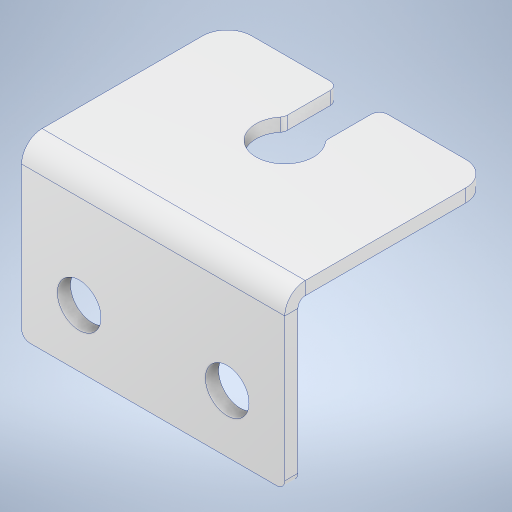
# Autodesk Inventor part: Door Stop
Saved by Autodesk Inventor 2024 (Build 280153000, 153)
## iProperties
Created: 2023-06-16
Part Number: Door Stop
Material: Aluminum 6061
Document SubType Name: Sheet Metal
Designer: Ishaan
Density: 2.7 g/cm^3
Appearance: Aluminum - Flat
Sheet Metal Rule: SendCutSend_Alu_1-16
Author: Ishaan
Autodesk Inventor part; units mm, degrees
ref_plane "YZ Plane" through (0, 0, 0) normal (1, 0, 0) x (0, 1, 0)
ref_plane "XZ Plane" through (0, 0, 0) normal (0, 1, 0) x (-1, 0, 0)
ref_plane "XY Plane" through (0, 0, 0) normal (0, 0, 1) x (1, 0, 0)
sketch "Sketch1" plane through (0, 0, 0) normal (0, 0, 1) x (1, 0, 0)
  line L0 (16, -7) -> (-16, -7)
  line L1 (-16, -7) -> (-16, 7)
  line L2 (-16, 7) -> (16, 7)
  line L3 (16, 7) -> (16, -7)
  line L4 (16, -7) -> (-16, 7) construction
  line L5 (-16, -7) -> (16, 7) construction
  line L6 (-9, 0) -> (9, 0) construction
  line L7 (-16, 7) -> (16, 7)
  line L8 (16, 7) -> (16, 12.25)
  line L9 (16, 12.25) -> (-16, 12.25)
  line L10 (-16, 12.25) -> (-16, 7)
  point P0 (0, 0)
  dimension "d126" = 32
  dimension "d127" = 14
  dimension "d128" = 7
  dimension "d129" = 12.25
  constraints: 22 end point, 4 parallel, 3 horizontal, 3 midpoint, 2 coincident, 2 perpendicular, 1 collinear
  measures "d126" distance of L1.end L2.end
  measures "d127" distance of L0.end L1.end
  measures "d128" distance from line of L6.start L1
  measures "d129" distance between parallel lines of L9 L6
extrude "Plate4" add sketch "Sketch1" along normal blind 1.6002
fillet "Fillet7" radius 1 2 edges at (16, -7, 0.8001) (-16, -7, 0.8001)
hole "Hole4" at (-9, 0, 0) at (9, 0, 0) direction (0, 0, 1) diameter 5.3 end through all
sketch "Sketch10" plane through (16, 12.25, 0) normal (0, 1, 0) x (-1, 0, 0)
  line L0 (32, 0) -> (0, 0)
  line L1 (0, 0) -> (0, -23.3998)
  line L2 (0, -23.3998) -> (32, -23.3998)
  line L3 (32, -23.3998) -> (32, 0)
  constraints: 6 end point, 1 horizontal, 1 perpendicular, 1 vertical
edge flange "Flange5" height 25 angle 90 thickness 1.6002 bend radius 0.889 thickness toward (0, 1, 0) relief tear relief width 1.6002 relief depth 0.8001 edges at (0, 12.25, 0) wall of the first edge with corners at (-16, 12.25, 0) (16, 12.25, 0) (16, 12.25, -23.3998) (-16, 12.25, -23.3998)
bend "Bend5"
corner "Corner5"
fillet "Fillet8" radius 3 2 edges at (16, 13.0501, -23.3998) (-16, 13.0501, -23.3998)
sketch "Sketch11" plane through (-16, 13.8502, -0.889) normal (0, 1, 0) x (1, 0, 0)
  arc A0 (32, 19.5108) -> (29, 22.5108) centre (29, 19.5108) ccw projected
  line L0 (3, 22.5108) -> (29, 22.5108) projected
  arc A1 (3, 22.5108) -> (0, 19.5108) centre (3, 19.5108) ccw projected
  line L1 (0, 0) -> (0, 19.5108) projected
  line L2 (0, 0) -> (32, 0) projected
  line L3 (32, 19.5108) -> (32, 0) projected
  circle A2 centre (16, 13.5108) radius 3.5
  line L4 (13.5, 22.5108) -> (18.5, 22.5108)
  line L5 (18.5, 22.5108) -> (18.5, 15.9603)
  line L6 (18.5, 15.9603) -> (13.5, 15.9603)
  line L7 (13.5, 15.9603) -> (13.5, 22.5108)
  point P0 (16, -0.889)
  point P1 (16, 22.5108)
  dimension "d149" = 7
  dimension "d150" = 9
  dimension "d151" = 5
  constraints: 8 end point, 2 midpoint, 2 parallel, 2 point on circle, 1 centre point, 1 horizontal, 1 perpendicular, 1 point on line
  measures "d149" diameter of A2
  measures "d150" distance from line of L0 A2.centre
  measures "d151" distance between parallel lines of L7 L5
extrude "Extrusion7" cut sketch "Sketch11" against normal through all contours L5 A2 L7 L0 | L6 A2 | A2 L6
fillet "Fillet9" radius 1 2 edges at (-2.5, 13.0501, -16.8493) (2.5, 13.0501, -16.8493)
fillet "Fillet10" radius 1 2 edges at (-2.5, 13.0501, -23.3998) (2.5, 13.0501, -23.3998)
equation "\"d71\" = Thickness"
equation "\"BendReliefWidth\" = Thickness"
equation "\"BendReliefDepth\" = 0.5 * Thickness"
equation "\"CornerReliefSize\" = 4 * Thickness"
equation "\"MinimumRemnant\" = 2 * Thickness"
equation "\"TransitionRadius\" = BendRadius"
equation "\"JacobiRadiusSize\" = BendRadius"
equation "\"GapSize\" = Thickness"
equation "\"Thickness\" = 1.6002"
equation "\"BendRadius\" = 0.889"
body "Solid2"
